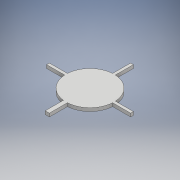
# Autodesk Inventor part: Zamek_II_klucz
Saved by Autodesk Inventor 2018 (Build 220112000, 112)
## iProperties
Created: 2018-10-19
Part Number: Zamek_II_klucz
Material: Ogólny
Document SubType Name: Modeling
Designer: EWA
Density: 1 g/cm^3
Appearance: Domyślna
Author: EWA
Autodesk Inventor part; units mm, degrees
ref_plane "YZ Plane" through (0, 0, 0) normal (1, 0, 0) x (0, 1, 0)
ref_plane "XZ Plane" through (0, 0, 0) normal (0, 1, 0) x (-1, 0, 0)
ref_plane "XY Plane" through (0, 0, 0) normal (0, 0, 1) x (1, 0, 0)
sketch "Szkic1" plane through (0, 0, 0) normal (0, 0, 1) x (1, 0, 0)
  circle A0 centre (0, 0) radius 43.5 construction
  line L0 (0, 43.5) -> (2.5, 43.5) construction
  line L1 (2.5, 43.5) -> (2.5, 75.9975) construction
  line L2 (2.5, 75.9975) -> (0, 75.9975) construction
  line L3 (0, 75.9975) -> (0, 43.5) construction
  line L4 (0, -43.5) -> (2.5, -43.5) construction
  line L5 (2.5, -43.5) -> (2.5, -75.9975) construction
  line L6 (2.5, -75.9975) -> (0, -75.9975) construction
  line L7 (43.5, 0) -> (75.9975, 0) construction
  line L8 (75.9975, 0) -> (75.9975, 2.5) construction
  line L9 (75.9975, 2.5) -> (43.5, 2.5) construction
  line L10 (43.5, 2.5) -> (43.5, 0) construction
  line L11 (43.5, 0) -> (75.9975, 0) construction
  line L12 (75.9975, 0) -> (75.9975, -2.5) construction
  line L13 (75.9975, -2.5) -> (43.5, -2.5) construction
  line L14 (43.5, -2.5) -> (43.5, 0) construction
  line L15 (0, 43.5) -> (-2.5, 43.5) construction
  line L16 (-2.5, 43.5) -> (-2.5, 75.9975) construction
  line L17 (-2.5, 75.9975) -> (0, 75.9975) construction
  line L18 (0, 75.9975) -> (0, 43.5) construction
  line L19 (0, -43.5) -> (-5, -43.5) construction
  line L20 (-5, -43.5) -> (-5, -75.9975) construction
  line L21 (-5, -75.9975) -> (-2.5, -75.9975) construction
  line L22 (-43.5, 0) -> (-75.9975, 0) construction
  line L23 (-75.9975, 0) -> (-75.9975, -2.5) construction
  line L24 (-75.9975, -2.5) -> (-43.5, -2.5) construction
  line L25 (-43.5, -2.5) -> (-43.5, 0) construction
  line L26 (-43.5, 0) -> (-75.9975, 0) construction
  line L27 (-75.9975, 0) -> (-75.9975, 2.5) construction
  line L28 (-75.9975, 2.5) -> (-43.5, 2.5) construction
  line L29 (-43.5, 2.5) -> (-43.5, 0) construction
  arc A1 (2.5, -43.4281) -> (43.4281, -2.5) centre (0, 0) ccw
  arc A2 (43.4281, 2.5) -> (2.5, 43.4281) centre (0, 0) ccw
  arc A3 (-43.4281, -2.5) -> (-5, -43.2117) centre (0, 0) ccw
  arc A4 (-2.5, 43.4281) -> (-43.4281, 2.5) centre (0, 0) ccw
  line L30 (-2.5, 43.4281) -> (-2.5, 75.9975)
  line L31 (-2.5, 75.9975) -> (2.5, 75.9975)
  line L32 (2.5, 75.9975) -> (2.5, 43.4281)
  line L33 (43.4281, 2.5) -> (75.9975, 2.5)
  line L34 (75.9975, 2.5) -> (75.9975, -2.5)
  line L35 (75.9975, -2.5) -> (43.4281, -2.5)
  line L36 (2.5, -43.4281) -> (2.5, -75.9975)
  line L37 (2.5, -75.9975) -> (-5, -75.9975)
  line L38 (-5, -75.9975) -> (-5, -43.2117)
  line L39 (-43.4281, -2.5) -> (-75.9975, -2.5)
  line L40 (-75.9975, -2.5) -> (-75.9975, 2.5)
  line L41 (-75.9975, 2.5) -> (-43.4281, 2.5)
  dimension "d0" = 87
  dimension "d1" = 2.5
  dimension "d3" = 2.5
  dimension "d6" = 2.5
  dimension "d7" = 2.5
  dimension "d8" = 2.5
  dimension "d9" = 2.5
  dimension "d11" = 2.5
  dimension "d12" = 2.5
  dimension "d15" = 75.9975
  dimension "d16" = 75.9975
  dimension "d17" = 75.9975
  dimension "d19" = 75.9975
  constraints: 84 end point, 14 parallel, 11 perpendicular, 8 collinear, 8 horizontal, 8 point on circle, 4 centre point, 4 point on line, 1 coincident, 18 other
  measures "d1" distance of L2.end L1.end
  measures "d3" distance of L5.end L6.end
  measures "d6" distance of L8.end L7.end
  measures "d7" distance of L11.end L12.end
  measures "d8" distance of L16.end L17.end
  measures "d9" distance of L21.end L20.end
  measures "d11" distance of L23.end L22.end
  measures "d12" distance of L26.end L27.end
  measures "d15" distance of L7.end point (0, 0)
  measures "d16" distance of L22.end point (0, 0)
  measures "d17" distance of L2.end point (0, 0)
  measures "d19" distance of L6.end point (0, 0)
extrude "Wyciągnięcie proste1" add sketch "Szkic1" along normal blind 6
equation "\"d1\" = d11"
equation "\"d3\" = d11"
equation "\"d6\" = d11"
equation "\"d7\" = d11"
equation "\"d8\" = d11"
equation "\"d9\" = d11"
equation "\"d12\" = d11"
equation "\"d16\" = d15"
equation "\"d17\" = d15"
equation "\"d19\" = d15"
